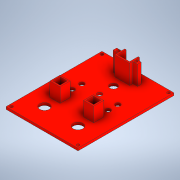
# Autodesk Inventor part: Lock
Saved by Autodesk Inventor 2021 (Build 250183000, 183)
## iProperties
Created: 2025-01-23
Part Number: Lock
Material: Generic
Document SubType Name: Modeling
Designer: User
Density: 1 g/cm^3
Appearance: Default
Author: User
Autodesk Inventor part; units mm, degrees
ref_plane "YZ Plane" through (0, 0, 0) normal (1, 0, 0) x (0, 1, 0)
ref_plane "XZ Plane" through (0, 0, 0) normal (0, 1, 0) x (-1, 0, 0)
ref_plane "XY Plane" through (0, 0, 0) normal (0, 0, 1) x (1, 0, 0)
sketch "Sketch1" plane through (0, 0, 0) normal (0, 1, 0) x (-1, 0, 0)
  line L0 (-75, 0) -> (-75, -100)
  line L1 (-75, -100) -> (75, -100)
  line L2 (75, -100) -> (75, 100)
  line L3 (75, 100) -> (-75, 100)
  line L4 (-75, 100) -> (-75, 0)
  circle A0 centre (69.4334, -94.4056) radius 3
  circle A1 centre (-69.396, -94.4056) radius 3
  circle A2 centre (-69.396, 94.4107) radius 3
  circle A3 centre (69.4334, 94.4107) radius 3
  point P0 (0, 0)
  dimension "d3" = 150
  dimension "d4" = 200
  dimension "d5" = 6
  dimension "d8" = 6
  dimension "d10" = 6
  dimension "d12" = 6
  constraints: 10 end point, 4 centre point, 4 perpendicular, 1 point on line
  measures "d3" distance of L0.end L1.end
  measures "d4" distance of L1.end L2.end
  measures "d5" diameter of A0
  measures "d8" diameter of A1
  measures "d10" diameter of A2
  measures "d12" diameter of A3
extrude "Extrusion1" add sketch "Sketch1" along normal blind 5
sketch "Sketch2" plane through (0, 5, 0) normal (0, 1, 0) x (1, 0, 0)
  circle A0 centre (-34.9985, -59.8752) radius 10
  circle A1 centre (35, -59.8759) radius 10
  line L0 (-35.1169, -34.8759) -> (-27.6169, -34.8759)
  line L1 (-27.6169, -34.8759) -> (-27.6169, -19.8759)
  line L2 (-27.6169, -19.8759) -> (-42.6169, -19.8759)
  line L3 (-42.6169, -19.8759) -> (-42.6169, -34.8759)
  line L4 (-42.6169, -34.8759) -> (-35.1169, -34.8759)
  line L5 (-27.6169, -37.8759) -> (-45.6169, -37.8759)
  line L6 (-45.6169, -37.8759) -> (-45.6169, -16.8759)
  line L7 (-45.6169, -16.8759) -> (-24.6169, -16.8759)
  line L8 (-24.6169, -16.8759) -> (-24.6169, -37.8759)
  line L9 (-24.6169, -37.8759) -> (-27.6169, -37.8759)
  line L10 (35, -34.8759) -> (42.5, -34.8759)
  line L11 (42.5, -34.8759) -> (42.5, -19.8759)
  line L12 (42.5, -19.8759) -> (27.5, -19.8759)
  line L13 (27.5, -19.8759) -> (27.5, -34.8759)
  line L14 (27.5, -34.8759) -> (35, -34.8759)
  line L15 (42.5, -37.8759) -> (24.5, -37.8759)
  line L16 (24.5, -37.8759) -> (24.5, -16.8759)
  line L17 (24.5, -16.8759) -> (45.5, -16.8759)
  line L18 (45.5, -16.8759) -> (45.5, -37.8759)
  line L19 (45.5, -37.8759) -> (42.5, -37.8759)
  line L20 (0, 85) -> (12.4518, 85)
  line L21 (12.4518, 85) -> (12.4518, 70)
  line L22 (12.4518, 70) -> (-12.5482, 70)
  line L23 (-12.5482, 70) -> (-12.5482, 85)
  line L24 (-12.5482, 85) -> (-0.0482, 85)
  line L25 (-12.5482, 85) -> (-12.5482, 77.5)
  circle A2 centre (-0.0482, 20) radius 6.5
  circle A3 centre (38, 20) radius 6.5
  line L26 (-75, 20) -> (-45, 20)
  circle A4 centre (-38.8669, 20) radius 6.5
  line L27 (12.4518, 67) -> (-15.5449, 67)
  line L28 (-15.5449, 67) -> (-15.5449, 88)
  line L29 (-15.5449, 88) -> (15.4551, 88)
  line L30 (15.4551, 88) -> (15.4551, 67)
  line L31 (15.4551, 67) -> (12.4518, 67)
  circle A5 centre (-18.5444, 77.4989) radius 3
  line L32 (-15.5449, 81.25) -> (-25.5449, 81.25)
  line L33 (-25.5449, 81.25) -> (-25.5449, 73.6405)
  line L34 (-25.5449, 73.6405) -> (-15.5449, 73.6405)
  circle A6 centre (18.4402, 77.4452) radius 3
  line L35 (15.4551, 73.6402) -> (25.4551, 73.6402)
  line L36 (25.4551, 73.6402) -> (25.4551, 81.25)
  line L37 (25.4551, 81.25) -> (15.4551, 81.25)
  line L38 (-12.5482, 85) -> (-15.5449, 85)
  line L39 (12.4518, 85) -> (15.4551, 85)
  line L40 (-12.5482, 85) -> (-12.5482, 88)
  line L41 (-12.5482, 70) -> (-12.5482, 67)
  line L42 (12.4518, 85) -> (12.4518, 88)
  line L43 (12.4518, 70) -> (12.4518, 67)
  line L44 (12.4518, 70) -> (15.4551, 70)
  line L45 (-12.5482, 70) -> (-15.5449, 70)
  point P0 (0, 0)
  point P1 (15.4551, 77.1464)
  point P2 (15.4551, 77.7441)
  point P3 (-15.5449, 77.5524)
  point P4 (-15.5449, 77.4455)
  dimension "d18" = 20
  dimension "d22" = 20
  dimension "d31" = 15
  dimension "d32" = 15
  dimension "d35" = 21
  dimension "d36" = 21
  dimension "d39" = 15
  dimension "d40" = 15
  dimension "d42" = 21
  dimension "d45" = 15
  dimension "d46" = 25
  dimension "d53" = 13
  dimension "d54" = 13
  dimension "d56" = 30
  dimension "d57" = 13
  dimension "d60" = 21
  dimension "d61" = 31
  dimension "d62" = 6
  dimension "d64" = 10
  dimension "d67" = 6
  dimension "d69" = 10
  constraints: 92 end point, 30 perpendicular, 19 point on line, 7 centre point, 7 horizontal, 1 collinear, 1 midpoint
  measures "d18" diameter of A0
  measures "d22" diameter of A1
  measures "d31" distance of L0.end L1.end
  measures "d32" distance of L1.end L2.end
  measures "d35" distance of L5.end L6.end
  measures "d36" distance of L6.end L7.end
  measures "d39" distance of L10.end L11.end
  measures "d40" distance of L11.end L12.end
  measures "d42" distance of L16.end L17.end
  measures "d45" distance of L20.end L21.end
  measures "d46" distance of L21.end L22.end
  measures "d53" diameter of A2
  measures "d54" diameter of A3
  measures "d56" distance of L26.start L26.end
  measures "d57" diameter of A4
  measures "d60" distance of L27.end L28.end
  measures "d61" distance of L28.end L29.end
  measures "d62" diameter of A5
  measures "d64" distance of L32.start L32.end
  measures "d67" diameter of A6
  measures "d69" distance of L35.start L35.end
extrude "Extrusion2" add sketch "Sketch2" along normal blind 40 contours L42 L29 L30 L39
extrude "Extrusion3" add sketch "Sketch2" along normal blind 40 contours L39 L30 A6 L44 L21
extrude "Extrusion4" add sketch "Sketch2" along normal blind 40 contours L40 L38 L28 L29
extrude "Extrusion5" add sketch "Sketch2" along normal blind 40 contours L45 L28 L38 L23
extrude "Extrusion6" add sketch "Sketch2" along normal blind 40 contours L41 L27 L28 L45
extrude "Extrusion7" add sketch "Sketch2" along normal blind 40 contours L43 L27 L41 L22
extrude "Extrusion8" add sketch "Sketch2" along normal blind 40 contours L44 L30 L31 L43
extrude "Extrusion9" add sketch "Sketch2" along normal blind 40 contours L37 L36 L35 L30 A6
extrude "Extrusion10" add sketch "Sketch2" along normal blind 40 contours L34 L33 L32 L28
extrude "Extrusion11" add sketch "Sketch2" along normal blind 30 contours L5 L6 L7 L8 L9
extrude "Extrusion12" add sketch "Sketch2" along normal blind 30 contours L15 L16 L17 L18 L19
sketch "Sketch3" plane through (0, 5, 0) normal (0, 1, 0) x (1, 0, 0)
  circle A0 centre (-35, -59.8417) radius 10
  circle A1 centre (35, -60) radius 10
  circle A2 centre (0, 20) radius 5
  circle A3 centre (38, 20) radius 5
  circle A4 centre (-37, 20) radius 5
  circle A5 centre (0, 0) radius 5
  circle A6 centre (38, 0) radius 5
  circle A7 centre (-37, 0) radius 5
  dimension "d94" = 20
  dimension "d95" = 20
  dimension "d101" = 10
  dimension "d103" = 10
  dimension "d104" = 10
  dimension "d106" = 10
  dimension "d107" = 10
  dimension "d108" = 10
  constraints: 8 centre point, 1 coincident
  measures "d94" diameter of A0
  measures "d95" diameter of A1
  measures "d101" diameter of A2
  measures "d103" diameter of A3
  measures "d104" diameter of A4
  measures "d106" diameter of A5
  measures "d107" diameter of A6
  measures "d108" diameter of A7
hole "Hole1" at (-35, 5, 59.8417) direction (0, -1, 0) diameter 20 end through all
hole "Hole2" at (35, 5, 60) direction (0, -1, 0) diameter 20 end through all
hole "Hole3" at (-37, 5, 0) direction (0, -1, 0) diameter 10 end through all
hole "Hole4" at (-37, 5, -20) direction (0, -1, 0) diameter 10 end through all
hole "Hole5" at (0, 5, -20) direction (0, -1, 0) diameter 10 end through all
hole "Hole6" at (0, 5, 0) direction (0, -1, 0) diameter 10 end through all
hole "Hole7" at (38, 5, -20) direction (0, -1, 0) diameter 10 end through all
hole "Hole8" at (38, 5, 0) direction (0, -1, 0) diameter 10 end through all
sketch "Sketch4" plane through (0, 5, 0) normal (0, 1, 0) x (1, 0, 0)
  circle A0 centre (0, 49) radius 7.5
  point P0 (0, 0)
  dimension "d166" = 15
  constraints: 1 centre point
  measures "d166" diameter of A0
hole "Hole9" at (0, 5, -49) direction (0, -1, 0) diameter 15 end through all
body "Solid1"
